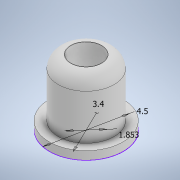
# Autodesk Inventor part: Lumipositor-WirePins
Saved by Autodesk Inventor 2022 (Build 260153000, 153)
## iProperties
Created: 2021-11-03
Part Number: Lumipositor-WirePins
Material: Generic
Document SubType Name: Modeling
Designer: incep
Density: 1 g/cm^3
Appearance: Default
Author: incep
Autodesk Inventor part; units mm, degrees
ref_plane "YZ Plane" through (0, 0, 0) normal (1, 0, 0) x (0, 1, 0)
ref_plane "XZ Plane" through (0, 0, 0) normal (0, 1, 0) x (-1, 0, 0)
ref_plane "XY Plane" through (0, 0, 0) normal (0, 0, 1) x (1, 0, 0)
sketch "Sketch1" plane through (0, 0, 0) normal (0, 1, 0) x (-1, 0, 0)
  circle A0 centre (0, 0) radius 0.9265
  circle A1 centre (0, 0) radius 1.7
  circle A2 centre (0, 0) radius 2.25
  dimension "d0" = 1.853
  dimension "d2" = 3.4
  dimension "d8" = 4.5
  constraints: 3 centre point, 2 coincident
  measures "d0" diameter of A0
  measures "d2" diameter of A1
  measures "d8" diameter of A2
sketch "Sketch2" plane through (0, 0, 0) normal (0, 1, 0) x (-1, 0, 0)
  circle A0 centre (0, 0) radius 1.193
  dimension "d3" = 2.386
  constraints: 1 centre point, 1 coincident
  measures "d3" diameter of A0
extrude "Extrusion1" add sketch "Sketch1" along normal blind 4 contours A1
extrude "Extrusion2" cut sketch "Sketch2" along normal blind 0.75
sketch "Sketch3" plane through (0, 0, 0) normal (0, -1, 0) x (1, 0, 0)
  point P0 (0, 0)
extrude "Extrusion3" add sketch "Sketch1" along normal blind 0.5 contours A2
fillet "Fillet1" radius 0.75 1 edges at (1.7, 4, 0)
body "Solid1"
